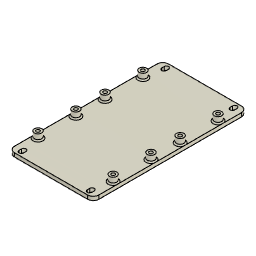
Lower Bay Tray - Dual LM2596 with LED (Autodesk Fusion 360 design; units mm, degrees)
Autodesk Fusion 360 part; units mm, degrees
note: some values were not read from the file. Set by a fixed rule: which sketch regions a step uses.
sketch "Sketch40" plane through (0, 0, 8) normal (0, 0, 1) x (1, 0, 0)
  circle A0 centre (65, 135) radius 1.4 construction
  circle A1 centre (65, 135) radius 3.4 construction
  circle A2 centre (10, 135) radius 1.4 construction
  circle A3 centre (10, 135) radius 3.4 construction
  circle A4 centre (-10, 135) radius 1.4 construction
  circle A5 centre (-10, 135) radius 3.4 construction
  circle A6 centre (-65, 135) radius 1.4 construction
  circle A7 centre (-65, 135) radius 3.4 construction
  circle A8 centre (-65, 20) radius 1.4 construction
  circle A9 centre (-65, 20) radius 3.4 construction
  circle A10 centre (-10, 20) radius 1.4 construction
  circle A11 centre (-10, 20) radius 3.4 construction
  circle A12 centre (10, 20) radius 1.4 construction
  circle A13 centre (10, 20) radius 3.4 construction
  circle A14 centre (65, 20) radius 1.4 construction
  circle A15 centre (65, 20) radius 3.4 construction
  line L0 (10, 135) -> (65, 135) construction
  line L1 (65, 135) -> (65, 20) construction
  line L2 (65, 20) -> (10, 20) construction
  line L3 (10, 20) -> (10, 135) construction
  line L4 (-10, 135) -> (-65, 135) construction
  line L5 (-65, 135) -> (-65, 20) construction
  line L6 (-65, 20) -> (-10, 20) construction
  line L7 (-10, 20) -> (-10, 135) construction
  arc A16 (-69.5, 20) -> (-65, 15.5) centre (-65, 20) ccw
  arc A17 (-10, 15.5) -> (-5.5, 20) centre (-10, 20) ccw
  arc A18 (-5.5, 135) -> (-10, 139.5) centre (-10, 135) ccw
  arc A19 (-65, 139.5) -> (-69.5, 135) centre (-65, 135) ccw
  line L8 (-69.5, 135) -> (-5.5, 135) construction
  line L9 (-5.5, 135) -> (-5.5, 20)
  line L10 (-10, 139.5) -> (-65, 139.5)
  line L11 (-10, 15.5) -> (-65, 15.5)
  line L12 (-69.5, 20) -> (-69.5, 135)
  line L13 (0, 0) -> (0, 50) construction
  line L14 (-66.8, 136) -> (-66.8, 134)
  arc A20 (-66.8, 134) -> (-63.2, 134) centre (-65, 134) ccw
  line L15 (-63.2, 134) -> (-63.2, 136)
  arc A21 (-63.2, 136) -> (-66.8, 136) centre (-65, 136) ccw
  line L16 (-65, 136) -> (-65, 134) construction
  arc A22 (-8.2, 136) -> (-11.8, 136) centre (-10, 136) ccw
  line L17 (-11.8, 136) -> (-11.8, 134)
  arc A23 (-11.8, 134) -> (-8.2, 134) centre (-10, 134) ccw
  line L18 (-8.2, 134) -> (-8.2, 136)
  line L19 (-5.5, 77.5) -> (-69.5, 77.5) construction
  arc A24 (-11.8, 19) -> (-8.2, 19) centre (-10, 19) ccw
  line L20 (-11.8, 19) -> (-11.8, 21)
  arc A25 (-8.2, 21) -> (-11.8, 21) centre (-10, 21) ccw
  line L21 (-8.2, 21) -> (-8.2, 19)
  arc A26 (-66.8, 19) -> (-63.2, 19) centre (-65, 19) ccw
  line L22 (-66.8, 19) -> (-66.8, 21)
  line L23 (-63.2, 21) -> (-63.2, 19)
  arc A27 (-63.2, 21) -> (-66.8, 21) centre (-65, 21) ccw
  line L24 (-37.5, 139.5) -> (-37.5, 15.5) construction
  point P0 (-65, 135)
  point P1 (-37.5, 77.5)
  dimension "d905" = 1.8
  dimension "d906" = 1.8
  dimension "d908" = 3.5
  dimension "d910" = 2
  dimension "d15" = 64
  constraint horizontal L0
  constraint vertical L1
  constraint horizontal L2
  constraint vertical L3
  constraint coincident A14.centre A15.centre
  constraint coincident A2.centre A3.centre
  constraint horizontal L4
  constraint vertical L5
  constraint horizontal L6
  constraint vertical L7
  constraint coincident A8.centre A9.centre
  constraint coincident A4.centre A5.centre
  constraint concentric A9 A16
  constraint concentric A11 A17
  constraint concentric A5 A18
  constraint concentric A7 A19
  constraint parallel L4 L8
  constraint tangent A17 L9
  constraint perpendicular L8 L9
  constraint tangent A19 L10
  constraint parallel L8 L10
  constraint tangent A16 L11
  constraint parallel L10 L11
  constraint tangent A19 L12
  constraint coincident L13.start origin
  constraint perpendicular L2 L13
  constraint tangent L14 A20
  constraint tangent A20 L15
  constraint parallel L14 L15
  constraint tangent L15 A21
  constraint tangent L14 A21
  constraint coincident L5 A20.centre
  constraint parallel L5 L16
  constraint coincident P0 A6.centre
  constraint midpoint L16 P0
  constraint tangent L17 A23
  constraint tangent A23 L18
  constraint parallel L17 L18
  constraint tangent A22 L18
  constraint tangent A22 L17
  constraint midpoint L9 L19.start
  constraint midpoint L12 L19.end
  constraint symmetric L14.start L19 A26.start
  constraint symmetric L14.end L19 L22.end
  constraint symmetric A20.end L19 L23.start
  constraint symmetric L15.end L19 A26.end
  constraint symmetric A20 L19 A27
  constraint symmetric A21 L19 A26
  constraint symmetric A22.end L19 A24.start
  constraint symmetric L17.end L19 L20.end
  constraint symmetric A22.start L19 A24.end
  constraint symmetric A23.end L19 A25.start
  constraint symmetric A22 L19 A24
  constraint symmetric A23 L19 A25
  constraint midpoint L10 L24.start
  constraint midpoint L11 L24.end
  constraint midpoint L24 P1
  constraint tangent A17 L11
  constraint tangent A16 L12
  constraint tangent A18 L10
  constraint tangent A18 L9
  measures "d905" radius of A21
  measures "d906" radius of A22
  measures "d908" distance of L10 A21.centre
  measures "d910" distance of A21.centre A20.centre
  measures "d15" distance of L9 L12
extrude "Extrude1" add sketch "Sketch40" along normal blind 3
move_face "OffsetFaces1" offset 2 2 faces at (-69.5, 58.3333, 9) (-5.5, 96.6667, 9)
sketch "Sketch1" plane through (0, 0, 11) normal (0, 0, 1) x (-1, 0, 0)
  arc A0 (63.2, -136) -> (66.8, -136) centre (65, -136) ccw
  line L0 (63.2, -136) -> (63.2, -134)
  arc A1 (66.8, -134) -> (63.2, -134) centre (65, -134) ccw
  line L1 (66.8, -134) -> (66.8, -136)
  arc A2 (66.8, -19) -> (63.2, -19) centre (65, -19) ccw
  line L2 (66.8, -19) -> (66.8, -21)
  arc A3 (63.2, -21) -> (66.8, -21) centre (65, -21) ccw
  line L3 (63.2, -21) -> (63.2, -19)
  line L4 (8.2, -136) -> (8.2, -134)
  arc A4 (11.8, -134) -> (8.2, -134) centre (10, -134) ccw
  line L5 (11.8, -134) -> (11.8, -136)
  arc A5 (8.2, -136) -> (11.8, -136) centre (10, -136) ccw
  arc A6 (11.8, -19) -> (8.2, -19) centre (10, -19) ccw
  line L6 (11.8, -19) -> (11.8, -21)
  arc A7 (8.2, -21) -> (11.8, -21) centre (10, -21) ccw
  line L7 (8.2, -21) -> (8.2, -19)
  arc A8 (8, -15.5) -> (3.5, -20) centre (8, -20) ccw
  line L8 (3.5, -20) -> (3.5, -135)
  arc A9 (3.5, -135) -> (8, -139.5) centre (8, -135) ccw
  line L9 (8, -139.5) -> (67, -139.5)
  arc A10 (67, -139.5) -> (71.5, -135) centre (67, -135) ccw
  line L10 (71.5, -135) -> (71.5, -20)
  arc A11 (71.5, -20) -> (67, -15.5) centre (67, -20) ccw
  line L11 (67, -15.5) -> (8, -15.5)
  line L12 (67.75, -89.25) -> (67.75, -119.75) construction
  line L13 (67.75, -119.75) -> (7.25, -119.75) construction
  line L14 (7.25, -119.75) -> (7.25, -89.25) construction
  line L15 (7.25, -89.25) -> (67.75, -89.25) construction
  line L16 (67.75, -89.25) -> (7.25, -119.75) construction
  line L17 (67.75, -119.75) -> (7.25, -89.25) construction
  circle A12 centre (7.25, -89.25) radius 1.4
  circle A13 centre (7.25, -119.75) radius 1.4
  circle A14 centre (67.75, -89.25) radius 1.4
  circle A15 centre (67.75, -119.75) radius 1.4
  circle A16 centre (67.75, -89.25) radius 3
  circle A17 centre (7.25, -89.25) radius 3
  circle A18 centre (7.25, -119.75) radius 3
  circle A19 centre (67.75, -119.75) radius 3
  line L18 (37.5, -104.5) -> (37.5, -139.5) construction
  line L19 (71.5, -77.5) -> (3.5, -77.5) construction
  circle A20 centre (67.75, -65.75) radius 3
  circle A21 centre (67.75, -65.75) radius 1.4
  circle A22 centre (67.75, -35.25) radius 1.4
  circle A23 centre (67.75, -35.25) radius 3
  circle A24 centre (7.25, -65.75) radius 3
  circle A25 centre (7.25, -65.75) radius 1.4
  circle A26 centre (7.25, -35.25) radius 1.4
  circle A27 centre (7.25, -35.25) radius 3
  point P0 (37.5, -104.5)
  dimension "d1" = 30.5
  dimension "d2" = 60.5
  dimension "d3" = 2.8
  dimension "d4" = 2.8
  dimension "d5" = 2.8
  dimension "d6" = 2.8
  dimension "d17" = 35
  dimension "d18" = 6
  dimension "d19" = 6
  dimension "d20" = 6
  dimension "d21" = 6
  constraint perpendicular L12 L13
  constraint parallel L12 L14
  constraint parallel L13 L15
  constraint coincident L16 P0
  constraint coincident L17 P0
  constraint coincident L14.end L15.start
  constraint coincident L13.end L14.start
  constraint coincident L12.start L15.end
  constraint coincident L12.end L13.start
  constraint coincident P0 L18.start
  constraint midpoint L9 L18.end
  constraint vertical L18
  constraint horizontal L13
  constraint concentric A15 A19
  constraint concentric A13 A18
  constraint concentric A14 A16
  constraint concentric A12 A17
  constraint midpoint L10 L19.start
  constraint midpoint L8 L19.end
  constraint symmetric A12 L19 A25
  constraint symmetric A13 L19 A26
  constraint symmetric A14 L19 A21
  constraint symmetric A15 L19 A22
  constraint symmetric A16 L19 A20
  constraint symmetric A17 L19 A24
  constraint symmetric A18 L19 A27
  constraint symmetric A19 L19 A23
  measures "d1" distance of L13.end L14.end
  measures "d2" distance of L12.end L13.end
  measures "d3" diameter of A12
  measures "d4" diameter of A13
  measures "d5" diameter of A14
  measures "d6" diameter of A15
  measures "d17" distance of P0 L18.end
  measures "d18" diameter of A16
  measures "d19" diameter of A17
  measures "d20" diameter of A18
  measures "d21" diameter of A19
extrude "Extrude2" add sketch "Sketch1" along normal blind 5 contours A16 | A17 | A18 | A19 | A20 | A23 | A24 | A27
fillet "Fillet1" radius 1 8 edges at (-4.453, 88.1652, 11) (-64.953, 88.1652, 11) (-4.453, 118.6652, 11) (-64.953, 118.6652, 11) (-64.953, 64.6652, 11) (-4.453, 64.6652, 11) (-4.453, 34.1652, 11) (-64.953, 34.1652, 11)
equation "d905 = large_m3 / 2"
equation "d906 = large_m3 / 2"
equation "large_m3 = 3.6 mm"
